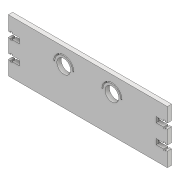
# Autodesk Inventor part: 2ureactor Torus
Saved by Autodesk Inventor 2018 (Build 220112000, 112)
## iProperties
Created: 2018-10-26
Part Number: 2ureactor Torus
Material: PPS Plastic
Document SubType Name: Modeling
Designer: mj.noguera10
Density: 1.637 g/cm^3
Appearance: Smooth - White
Author: mj.noguera10
Autodesk Inventor part; units mm, degrees
ref_plane "YZ Plane" through (0, 0, 0) normal (1, 0, 0) x (0, 1, 0)
ref_plane "XZ Plane" through (0, 0, 0) normal (0, 1, 0) x (-1, 0, 0)
ref_plane "XY Plane" through (0, 0, 0) normal (0, 0, 1) x (1, 0, 0)
sketch "Sombreado_1" plane through (0, 0, 0) normal (0, 0, 1) x (1, 0, 0)
  point P0 (0, 0)
sketch "Sombreado_2" plane through (0, 0, 0) normal (0, 0, 1) x (1, 0, 0)
  point P0 (0, 0)
sketch "Sombreado_3" plane through (0, 0, 0) normal (0, 0, 1) x (1, 0, 0)
  point P0 (0, 0)
sketch "Boceto1" plane through (0, 0, 0) normal (0, 1, 0) x (-1, 0, 0)
  line L0 (30.3882, 1.25) -> (30.8882, 1.25)
  line L1 (0, -6.75) -> (75, -6.75)
  line L2 (75, -6.75) -> (75, 18.25)
  line L3 (75, 18.25) -> (0, 18.25)
  line L4 (0, 18.25) -> (0, -6.75)
  arc A0 (21.3882, 1.25) -> (30.8882, 1.25) centre (26.1382, 1.25) ccw
  arc A1 (21.8882, 1.25) -> (30.3882, 1.25) centre (26.1382, 1.25) ccw
  line L5 (21.3882, 1.25) -> (21.8882, 1.25)
  line L6 (1.8, 2.5) -> (5.3, 2.5)
  line L7 (1.8, 2.5) -> (1.8, 3)
  line L8 (1.8, 3) -> (1, 3)
  line L9 (1, 3) -> (1, 2.5)
  line L10 (1, 0) -> (0, 0)
  line L11 (1, 0) -> (1, -0.5)
  line L12 (1, -0.5) -> (1.8, -0.5)
  line L13 (1.8, -0.5) -> (1.8, 0)
  line L14 (5.3, 0) -> (1.8, 0)
  line L15 (0, 2.5) -> (1, 2.5)
  line L16 (1.8, 11.5) -> (5.3, 11.5)
  line L17 (5.3, 9) -> (1.8, 9)
  line L18 (1, 9) -> (0, 9)
  line L19 (0, 11.5) -> (1, 11.5)
  line L20 (1.8, 11.5) -> (1.8, 12)
  line L21 (1.8, 12) -> (1, 12)
  line L22 (1, 12) -> (1, 11.5)
  line L23 (1, 9) -> (1, 8.5)
  line L24 (1, 8.5) -> (1.8, 8.5)
  line L25 (1.8, 8.5) -> (1.8, 9)
  line L26 (44.6082, 1.25) -> (44.1082, 1.25)
  arc A2 (44.1082, 1.25) -> (53.6082, 1.25) centre (48.8582, 1.25) ccw
  arc A3 (44.6082, 1.25) -> (53.1082, 1.25) centre (48.8582, 1.25) ccw
  line L27 (53.6082, 1.25) -> (53.1082, 1.25)
  line L28 (73.1964, 2.5) -> (69.6964, 2.5)
  line L29 (69.6964, 0) -> (73.1964, 0)
  line L30 (73.9964, 0) -> (74.9964, 0)
  line L31 (74.9964, 2.5) -> (73.9964, 2.5)
  line L32 (73.1964, 2.5) -> (73.1964, 3)
  line L33 (73.1964, 3) -> (73.9964, 3)
  line L34 (73.9964, 3) -> (73.9964, 2.5)
  line L35 (73.9964, 0) -> (73.9964, -0.5)
  line L36 (73.9964, -0.5) -> (73.1964, -0.5)
  line L37 (73.1964, -0.5) -> (73.1964, 0)
  line L38 (73.1964, 11.5) -> (69.6964, 11.5)
  line L39 (69.6964, 9) -> (73.1964, 9)
  line L40 (73.9964, 9) -> (74.9964, 9)
  line L41 (74.9964, 11.5) -> (73.9964, 11.5)
  line L42 (73.1964, 11.5) -> (73.1964, 12)
  line L43 (73.1964, 12) -> (73.9964, 12)
  line L44 (73.9964, 12) -> (73.9964, 11.5)
  line L45 (73.9964, 9) -> (73.9964, 8.5)
  line L46 (73.9964, 8.5) -> (73.1964, 8.5)
  line L47 (73.1964, 8.5) -> (73.1964, 9)
  line L48 (75, 18.25) -> (75, 43.25)
  line L49 (75, 43.25) -> (0, 43.25)
  line L50 (0, 43.25) -> (0, 18.25)
  line L51 (5.3, 11.5) -> (5.3, 9)
  line L52 (5.3, 2.5) -> (5.3, 0)
  line L53 (69.6964, 11.5) -> (69.6964, 9)
  line L54 (69.6964, 2.5) -> (69.6964, 0)
  circle A4 centre (26.1382, 1.25) radius 3.25
  circle A5 centre (48.8582, 1.25) radius 3.25
  circle A6 centre (26.1382, 26.25) radius 3.25
  circle A7 centre (48.8582, 26.25) radius 3.25
  line L55 (75, 43.25) -> (75, 68.25)
  line L56 (75, 68.25) -> (0, 68.25)
  line L57 (0, 68.25) -> (0, 43.25)
  circle A8 centre (26.1382, 51.25) radius 3.25
  circle A9 centre (48.8582, 51.25) radius 3.25
  point P0 (0, 0)
  constraints: 116 end point, 10 centre point, 8 point on circle
sketch "Boceto3" plane through (0, 0, 0) normal (0, 1, 0) x (-1, 0, 0)
  line L0 (0, 0) -> (-75, 0)
  line L1 (-75, 0) -> (-75, -25)
  line L2 (-75, -25) -> (0, -25)
  line L3 (0, -25) -> (0, 0)
  line L4 (0, 0) -> (-75, 0)
  line L5 (-75, 0) -> (-75, -25)
  line L6 (-75, -25) -> (0, -25)
  line L7 (0, -25) -> (0, 0)
  dimension "d4" = 75
  dimension "d5" = 25
  dimension "d6" = 75
  dimension "d7" = 25
  constraints: 16 end point, 4 parallel, 2 horizontal, 2 perpendicular
  measures "d4" distance of L2.end L1.end
  measures "d5" distance of L1.end L1.start
  measures "d6" distance of L6.end L5.end
  measures "d7" distance of L5.end L5.start
extrude "Extrusión1" add sketch "Boceto3" along normal blind 2
sketch "Boceto4" plane through (0, 2, 0) normal (0, 1, 0) x (1, 0, 0)
  line L0 (-1.8065, 18.25) -> (1.0036, 18.25)
  line L1 (-1.8065, 15.75) -> (1.0036, 15.75)
  line L2 (1.0036, 15.75) -> (1.0036, 15.25)
  line L3 (1.8036, 15.75) -> (1.8036, 15.25)
  line L4 (1.0036, 18.75) -> (1.8036, 18.75)
  line L5 (1.0036, 15.25) -> (1.8036, 15.25)
  line L6 (1.0036, 18.25) -> (1.0036, 18.75)
  line L7 (1.8036, 18.75) -> (1.8036, 18.25)
  line L8 (1.8036, 18.25) -> (5.3036, 18.25)
  line L9 (1.8036, 15.75) -> (5.3036, 15.75)
  line L10 (5.3036, 18.25) -> (5.3036, 15.75)
  line L11 (-1.5403, 9.25) -> (-1.5403, 6.75)
  line L12 (-1.5403, 9.25) -> (1.0036, 9.25)
  line L13 (-1.5403, 6.75) -> (1.0036, 6.75)
  line L14 (1.0036, 6.75) -> (1.0036, 6.25)
  line L15 (1.8036, 6.75) -> (1.8036, 6.25)
  line L16 (1.0036, 9.75) -> (1.8036, 9.75)
  line L17 (1.0036, 6.25) -> (1.8036, 6.25)
  line L18 (1.0036, 9.25) -> (1.0036, 9.75)
  line L19 (1.8036, 9.75) -> (1.8036, 9.25)
  line L20 (1.8036, 9.25) -> (5.3036, 9.25)
  line L21 (1.8036, 6.75) -> (5.3036, 6.75)
  line L22 (5.3036, 9.25) -> (5.3036, 6.75)
  circle A0 centre (26.1418, 8) radius 3.25
  arc A1 (21.3918, 8) -> (30.8918, 8) centre (26.1418, 8) ccw
  arc A2 (21.8918, 8) -> (30.3918, 8) centre (26.1418, 8) ccw
  line L23 (30.3918, 8) -> (30.8918, 8)
  line L24 (21.8918, 8) -> (21.3918, 8)
  line L25 (-1.8065, 18.25) -> (-1.8065, 15.75)
  line L26 (5.3036, 15.75) -> (7.3036, 16.75)
  line L27 (5.3036, 18.25) -> (7.3036, 17.25)
  line L28 (7.3036, 16.75) -> (9.4436, 16.75)
  line L29 (9.4436, 16.75) -> (13.6836, 12.5)
  line L30 (9.7963, 17.1027) -> (9.7972, 17.1036)
  line L31 (14.1397, 12.749) -> (9.6494, 17.25)
  line L32 (7.3036, 17.25) -> (9.6494, 17.25)
  line L33 (5.3036, 9.25) -> (7.3036, 8.25)
  line L34 (5.3036, 6.75) -> (7.3036, 7.75)
  line L35 (7.3036, 8.25) -> (9.4436, 8.25)
  line L36 (9.4436, 8.25) -> (13.6836, 12.5)
  line L37 (14.1397, 12.251) -> (9.6494, 7.75)
  line L38 (7.3036, 7.75) -> (9.6494, 7.75)
  line L39 (14.1397, 12.749) -> (26.1418, 12.749)
  line L40 (14.1397, 12.251) -> (26.1418, 12.251)
  arc A3 (30.3918, 8) -> (26.1418, 12.25) centre (26.1418, 8) ccw
  arc A4 (30.8918, 8) -> (26.1418, 12.75) centre (26.1418, 8) ccw
  line L41 (0, 0) -> (75, 0) projected
  line L42 (75, 25) -> (0, 25) projected
  line L43 (76.8065, 18.25) -> (73.9964, 18.25)
  line L44 (76.8065, 15.75) -> (73.9964, 15.75)
  line L45 (73.9964, 15.75) -> (73.9964, 15.25)
  line L46 (73.1964, 15.75) -> (73.1964, 15.25)
  line L47 (73.9964, 18.75) -> (73.1964, 18.75)
  line L48 (73.9964, 15.25) -> (73.1964, 15.25)
  line L49 (73.9964, 18.25) -> (73.9964, 18.75)
  line L50 (73.1964, 18.75) -> (73.1964, 18.25)
  line L51 (73.1964, 18.25) -> (69.6964, 18.25)
  line L52 (73.1964, 15.75) -> (69.6964, 15.75)
  line L53 (69.6964, 18.25) -> (69.6964, 15.75)
  line L54 (69.6964, 9.25) -> (69.6964, 6.75)
  line L55 (73.1964, 6.75) -> (73.1964, 6.25)
  line L56 (73.1964, 6.75) -> (69.6964, 6.75)
  line L57 (73.1964, 9.75) -> (73.1964, 9.25)
  line L58 (73.9964, 6.75) -> (73.9964, 6.25)
  line L59 (73.9964, 6.25) -> (73.1964, 6.25)
  line L60 (73.9964, 9.75) -> (73.1964, 9.75)
  line L61 (73.9964, 9.25) -> (73.9964, 9.75)
  line L62 (76.5403, 9.25) -> (76.5403, 6.75)
  line L63 (76.5403, 9.25) -> (73.9964, 9.25)
  line L64 (76.5403, 6.75) -> (73.9964, 6.75)
  line L65 (73.1964, 9.25) -> (69.6964, 9.25)
  circle A5 centre (48.8582, 8) radius 3.25
  arc A6 (44.1082, 8) -> (53.6082, 8) centre (48.8582, 8) ccw
  arc A7 (44.6082, 8) -> (53.1082, 8) centre (48.8582, 8) ccw
  line L66 (44.6082, 8) -> (44.1082, 8)
  line L67 (53.1082, 8) -> (53.6082, 8)
  line L68 (76.8065, 18.25) -> (76.8065, 15.75)
  line L69 (69.6964, 15.75) -> (67.6964, 16.75)
  line L70 (69.6964, 18.25) -> (67.6964, 17.25)
  line L71 (67.6964, 16.75) -> (65.5564, 16.75)
  line L72 (65.5564, 16.75) -> (61.3164, 12.5)
  line L73 (65.2037, 17.1027) -> (65.2028, 17.1036)
  line L74 (60.8603, 12.749) -> (65.3506, 17.25)
  line L75 (67.6964, 17.25) -> (65.3506, 17.25)
  line L76 (67.6964, 8.25) -> (65.5564, 8.25)
  line L77 (67.6964, 7.75) -> (65.3506, 7.75)
  line L78 (60.8603, 12.251) -> (65.3506, 7.75)
  line L79 (65.5564, 8.25) -> (61.3164, 12.5)
  line L80 (69.6964, 9.25) -> (67.6964, 8.25)
  line L81 (69.6964, 6.75) -> (67.6964, 7.75)
  line L82 (60.8603, 12.749) -> (48.8582, 12.749)
  line L83 (60.8603, 12.251) -> (48.8582, 12.251)
  arc A8 (48.8582, 12.25) -> (44.6082, 8) centre (48.8582, 8) ccw
  arc A9 (48.8582, 12.75) -> (44.1082, 8) centre (48.8582, 8) ccw
  constraints: 164 end point, 16 point on circle, 14 horizontal, 10 centre point, 8 coincident, 8 vertical, 4 parallel, 2 point on line, 1 perpendicular
extrude "Extrusión2" cut sketch "Boceto4" against normal blind 2 contours L0 L6 L4 L7 L8 L10 L9 L3 L5 L2 L1 L25 | A1 L24 A2 L23 | L22 L21 L15 L17 L14 L13 L11 L12 L18 L16 L19 L20 | A0 | L68 L44 L45 L48 L46 L52 L53 L51 L50 L47 L49 L43 | L66 A7 L67 A6 | L65 L57 L60 L61 L63 L62 L64 L58 L59 L55 L56 L54 | A5
sketch "Boceto5" plane through (0, 2, 0) normal (0, 1, 0) x (1, 0, 0)
  line L0 (5.3036, 18.25) -> (5.3036, 15.75)
  line L1 (5.3036, 9.25) -> (5.3036, 6.75)
  line L2 (5.3036, 15.75) -> (7.3036, 16.75)
  line L3 (5.3036, 18.25) -> (7.3036, 17.25)
  line L4 (7.3036, 16.75) -> (9.4436, 16.75)
  line L5 (9.4436, 16.75) -> (13.6836, 12.5)
  line L6 (9.7963, 17.1027) -> (9.7972, 17.1036)
  line L7 (14.1397, 12.749) -> (9.6494, 17.25)
  line L8 (7.3036, 17.25) -> (9.6494, 17.25)
  line L9 (7.3036, 8.25) -> (9.4436, 8.25)
  line L10 (7.3036, 7.75) -> (9.6494, 7.75)
  line L11 (14.1397, 12.251) -> (9.6494, 7.75)
  line L12 (9.4436, 8.25) -> (13.6836, 12.5)
  line L13 (5.3036, 9.25) -> (7.3036, 8.25)
  line L14 (5.3036, 6.75) -> (7.3036, 7.75)
  line L15 (14.1397, 12.749) -> (26.1418, 12.749)
  line L16 (14.1397, 12.251) -> (26.1418, 12.251)
  line L17 (30.8908, 8) -> (30.3928, 8)
  arc A0 (30.3928, 8) -> (26.1418, 12.251) centre (26.1418, 8) ccw
  arc A1 (30.8908, 8) -> (26.1418, 12.749) centre (26.1418, 8) ccw
  line L18 (69.6964, 18.25) -> (69.6964, 15.75)
  line L19 (69.6964, 9.25) -> (69.6964, 6.75)
  line L20 (69.6964, 15.75) -> (67.6964, 16.75)
  line L21 (69.6964, 18.25) -> (67.6964, 17.25)
  line L22 (67.6964, 16.75) -> (65.5564, 16.75)
  line L23 (65.5564, 16.75) -> (61.3164, 12.5)
  line L24 (65.2037, 17.1027) -> (65.2028, 17.1036)
  line L25 (60.8603, 12.749) -> (65.3506, 17.25)
  line L26 (67.6964, 17.25) -> (65.3506, 17.25)
  line L27 (67.6964, 8.25) -> (65.5564, 8.25)
  line L28 (67.6964, 7.75) -> (65.3506, 7.75)
  line L29 (60.8603, 12.251) -> (65.3506, 7.75)
  line L30 (65.5564, 8.25) -> (61.3164, 12.5)
  line L31 (69.6964, 9.25) -> (67.6964, 8.25)
  line L32 (69.6964, 6.75) -> (67.6964, 7.75)
  line L33 (60.8603, 12.749) -> (48.8582, 12.749)
  line L34 (60.8603, 12.251) -> (48.8582, 12.251)
  line L35 (44.1092, 8) -> (44.6072, 8)
  arc A2 (48.8582, 12.251) -> (44.6072, 8) centre (48.8582, 8) ccw
  arc A3 (48.8582, 12.749) -> (44.1092, 8) centre (48.8582, 8) ccw
  point P0 (0, 0)
  constraints: 72 end point, 8 point on circle, 4 centre point, 2 coincident, 2 horizontal, 2 point on line, 2 vertical
extrude "Extrusión3" cut sketch "Boceto5" against normal blind 1
